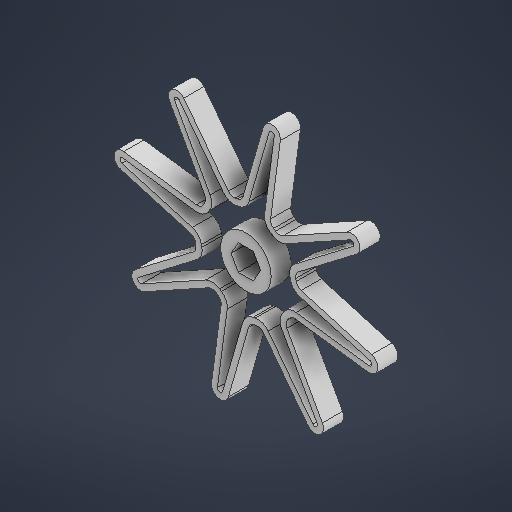
# Autodesk Inventor part: molde star
Saved by Autodesk Inventor 2025 (Build 290162010, 162A)
## iProperties
Created: 2025-01-06
Part Number: molde star
Material: Genérico
Document SubType Name: Modeling
Designer: Win-10
Density: 1 g/cm^3
Appearance: Padrão
Author: Win-10
Autodesk Inventor part; units mm, degrees
ref_plane "YZ Plane" through (0, 0, 0) normal (1, 0, 0) x (0, 1, 0)
ref_plane "XZ Plane" through (0, 0, 0) normal (0, 1, 0) x (-1, 0, 0)
ref_plane "XY Plane" through (0, 0, 0) normal (0, 0, 1) x (1, 0, 0)
sketch "Esboço1" plane through (0, 0, 0) normal (0, 0, 1) x (1, 0, 0)
  line L0 (51.4739, 35.1611) -> (19.7673, 17.6332) projected
  arc A0 (12.9851, 18.0371) -> (19.7673, 17.6332) centre (16.6951, 23.1906) ccw projected
  line L1 (12.9851, 18.0371) -> (12.0737, 18.6595) projected
  arc A1 (9.229, 24.8295) -> (12.0737, 18.6595) centre (15.5233, 23.9908) ccw projected
  line L2 (9.229, 24.8295) -> (14.0142, 60.741) projected
  arc A2 (14.0142, 60.741) -> (11.5349, 61.2602) centre (12.7553, 60.9087) ccw projected
  line L3 (11.5349, 61.2602) -> (1.509, 26.4462) projected
  arc A3 (-3.5723, 21.936) -> (1.509, 26.4462) centre (-4.593, 28.2035) ccw projected
  line L4 (-3.5723, 21.936) -> (-4.6569, 21.7316) projected
  arc A4 (-11.0312, 24.083) -> (-4.6569, 21.7316) centre (-5.9874, 27.9407) ccw projected
  line L5 (-11.0312, 24.083) -> (-33.0408, 52.8599) projected
  arc A5 (-33.0408, 52.8599) -> (-35.1611, 51.4739) centre (-34.0496, 52.0884) ccw projected
  line L6 (-35.1611, 51.4739) -> (-17.6332, 19.7673) projected
  arc A6 (-18.0371, 12.9851) -> (-17.6332, 19.7673) centre (-23.1906, 16.6951) ccw projected
  line L7 (-18.0371, 12.9851) -> (-18.6595, 12.0737) projected
  arc A7 (-24.8295, 9.229) -> (-18.6595, 12.0737) centre (-23.9908, 15.5233) ccw projected
  line L8 (-24.8295, 9.229) -> (-60.741, 14.0142) projected
  arc A8 (-60.741, 14.0142) -> (-61.2602, 11.5349) centre (-60.9087, 12.7553) ccw projected
  line L9 (-61.2602, 11.5349) -> (-26.4462, 1.509) projected
  arc A9 (-21.936, -3.5723) -> (-26.4462, 1.509) centre (-28.2035, -4.593) ccw projected
  line L10 (-21.936, -3.5723) -> (-21.7316, -4.6569) projected
  arc A10 (-24.083, -11.0312) -> (-21.7316, -4.6569) centre (-27.9407, -5.9874) ccw projected
  line L11 (-24.083, -11.0312) -> (-52.8599, -33.0408) projected
  arc A11 (-52.8599, -33.0408) -> (-51.4739, -35.1611) centre (-52.0884, -34.0496) ccw projected
  line L12 (-51.4739, -35.1611) -> (-19.7673, -17.6332) projected
  arc A12 (-12.9851, -18.0371) -> (-19.7673, -17.6332) centre (-16.6951, -23.1906) ccw projected
  line L13 (-12.9851, -18.0371) -> (-12.0737, -18.6595) projected
  arc A13 (-9.229, -24.8295) -> (-12.0737, -18.6595) centre (-15.5233, -23.9908) ccw projected
  line L14 (-9.229, -24.8295) -> (-14.0142, -60.741) projected
  arc A14 (-14.0142, -60.741) -> (-11.5349, -61.2602) centre (-12.7553, -60.9087) ccw projected
  line L15 (-11.5349, -61.2602) -> (-1.509, -26.4462) projected
  arc A15 (3.5723, -21.936) -> (-1.509, -26.4462) centre (4.593, -28.2035) ccw projected
  line L16 (3.5723, -21.936) -> (4.6569, -21.7316) projected
  arc A16 (11.0312, -24.083) -> (4.6569, -21.7316) centre (5.9874, -27.9407) ccw projected
  line L17 (11.0312, -24.083) -> (33.0408, -52.8599) projected
  arc A17 (33.0408, -52.8599) -> (35.1611, -51.4739) centre (34.0496, -52.0884) ccw projected
  line L18 (35.1611, -51.4739) -> (17.6332, -19.7673) projected
  arc A18 (18.0371, -12.9851) -> (17.6332, -19.7673) centre (23.1906, -16.6951) ccw projected
  line L19 (18.0371, -12.9851) -> (18.6595, -12.0737) projected
  arc A19 (24.8295, -9.229) -> (18.6595, -12.0737) centre (23.9908, -15.5233) ccw projected
  line L20 (24.8295, -9.229) -> (60.741, -14.0142) projected
  arc A20 (60.741, -14.0142) -> (61.2602, -11.5349) centre (60.9087, -12.7553) ccw projected
  line L21 (61.2602, -11.5349) -> (26.4462, -1.509) projected
  arc A21 (21.936, 3.5723) -> (26.4462, -1.509) centre (28.2035, 4.593) ccw projected
  line L22 (21.936, 3.5723) -> (21.7316, 4.6569) projected
  arc A22 (24.083, 11.0312) -> (21.7316, 4.6569) centre (27.9407, 5.9874) ccw projected
  line L23 (24.083, 11.0312) -> (52.8599, 33.0408) projected
  arc A23 (52.8599, 33.0408) -> (51.4739, 35.1611) centre (52.0884, 34.0496) ccw projected
  line L24 (54.6824, 30.6579) -> (25.9055, 8.6483)
  arc A24 (25.9055, 8.6483) -> (24.6718, 5.2548) centre (27.9407, 5.9874) ccw
  line L25 (24.6718, 5.2548) -> (24.8921, 4.0855)
  arc A25 (24.8921, 4.0855) -> (27.2764, 1.3738) centre (28.2035, 4.593) ccw
  line L26 (27.2764, 1.3738) -> (62.0904, -8.6521)
  arc A26 (60.3447, -16.9879) -> (62.0904, -8.6521) centre (60.9087, -12.7553) ccw
  line L27 (60.3447, -16.9879) -> (24.4332, -12.2027)
  arc A27 (24.4332, -12.2027) -> (21.1613, -13.7298) centre (23.9908, -15.5233) ccw
  line L28 (21.1613, -13.7298) -> (20.4903, -14.7125)
  arc A28 (20.4903, -14.7125) -> (20.2587, -18.3159) centre (23.1906, -16.6951) ccw
  line L29 (20.2587, -18.3159) -> (37.7866, -50.0225)
  arc A29 (30.6579, -54.6824) -> (37.7866, -50.0225) centre (34.0496, -52.0884) ccw
  line L30 (30.6579, -54.6824) -> (8.6483, -25.9055)
  arc A30 (8.6483, -25.9055) -> (5.2548, -24.6718) centre (5.9874, -27.9407) ccw
  line L31 (5.2548, -24.6718) -> (4.0855, -24.8921)
  arc A31 (4.0855, -24.8921) -> (1.3738, -27.2764) centre (4.593, -28.2035) ccw
  line L32 (1.3738, -27.2764) -> (-8.6521, -62.0904)
  arc A32 (-16.9879, -60.3447) -> (-8.6521, -62.0904) centre (-12.7553, -60.9087) ccw
  line L33 (-16.9879, -60.3447) -> (-12.2027, -24.4332)
  arc A33 (-12.2027, -24.4332) -> (-13.7298, -21.1613) centre (-15.5233, -23.9908) ccw
  line L34 (-13.7298, -21.1613) -> (-14.7125, -20.4903)
  arc A34 (-14.7125, -20.4903) -> (-18.3159, -20.2587) centre (-16.6951, -23.1906) ccw
  line L35 (-18.3159, -20.2587) -> (-50.0225, -37.7866)
  arc A35 (-54.6824, -30.6579) -> (-50.0225, -37.7866) centre (-52.0884, -34.0496) ccw
  line L36 (-54.6824, -30.6579) -> (-25.9055, -8.6483)
  arc A36 (-25.9055, -8.6483) -> (-24.6718, -5.2548) centre (-27.9407, -5.9874) ccw
  line L37 (-24.6718, -5.2548) -> (-24.8921, -4.0855)
  arc A37 (-24.8921, -4.0855) -> (-27.2764, -1.3738) centre (-28.2035, -4.593) ccw
  line L38 (-27.2764, -1.3738) -> (-62.0904, 8.6521)
  arc A38 (-60.3447, 16.9879) -> (-62.0904, 8.6521) centre (-60.9087, 12.7553) ccw
  line L39 (-60.3447, 16.9879) -> (-24.4332, 12.2027)
  arc A39 (-24.4332, 12.2027) -> (-21.1613, 13.7298) centre (-23.9908, 15.5233) ccw
  line L40 (-21.1613, 13.7298) -> (-20.4903, 14.7125)
  arc A40 (-20.4903, 14.7125) -> (-20.2587, 18.3159) centre (-23.1906, 16.6951) ccw
  line L41 (-20.2587, 18.3159) -> (-37.7866, 50.0225)
  arc A41 (-30.6579, 54.6824) -> (-37.7866, 50.0225) centre (-34.0496, 52.0884) ccw
  line L42 (-30.6579, 54.6824) -> (-8.6483, 25.9055)
  arc A42 (-8.6483, 25.9055) -> (-5.2548, 24.6718) centre (-5.9874, 27.9407) ccw
  line L43 (-5.2548, 24.6718) -> (-4.0855, 24.8921)
  arc A43 (-4.0855, 24.8921) -> (-1.3738, 27.2764) centre (-4.593, 28.2035) ccw
  line L44 (-1.3738, 27.2764) -> (8.6521, 62.0904)
  arc A44 (16.9879, 60.3447) -> (8.6521, 62.0904) centre (12.7553, 60.9087) ccw
  line L45 (16.9879, 60.3447) -> (12.2027, 24.4332)
  arc A45 (12.2027, 24.4332) -> (13.7298, 21.1613) centre (15.5233, 23.9908) ccw
  line L46 (13.7298, 21.1613) -> (14.7125, 20.4903)
  arc A46 (14.7125, 20.4903) -> (18.3159, 20.2587) centre (16.6951, 23.1906) ccw
  line L47 (18.3159, 20.2587) -> (50.0225, 37.7866)
  arc A47 (54.6824, 30.6579) -> (50.0225, 37.7866) centre (52.0884, 34.0496) ccw
  circle A48 centre (0, 0) radius 12.5
  line L48 (7.3323, 0) -> (3.6662, -6.35)
  line L49 (3.6662, -6.35) -> (-3.6662, -6.35)
  line L50 (-3.6662, -6.35) -> (-7.3323, 0)
  line L51 (-7.3323, 0) -> (-3.6662, 6.35)
  line L52 (-3.6662, 6.35) -> (3.6662, 6.35)
  line L53 (3.6662, 6.35) -> (7.3323, 0)
  dimension "d0" = 25
  dimension "d1" = 12.7
  dimension "d2" = 36.2289
  dimension "d3" = 4.27
  dimension "d4" = 3.35
  dimension "d6" = 3.6108
  dimension "d7" = 3.6108
  dimension "d8" = 3.6108
  dimension "d9" = 3.6108
  dimension "d10" = 3.6034
  dimension "d11" = 3.6108
  dimension "d12" = 3.6034
  constraints: 60 end point, 48 point on circle, 25 centre point, 23 equal length, 22 equal radius, 16 tangent, 2 coincident, 1 horizontal, 14 other
  measures "d0" diameter of A48
  measures "d1" distance between parallel lines of L49 L52
  measures "d2" distance of L42.start L42.end
  measures "d3" radius of A41
  measures "d4" radius of A42
  measures "d6" distance of L45.end L46.start
  measures "d7" distance of L24.end L25.start
  measures "d8" distance of L27.end L28.start
  measures "d9" distance of L30.end L31.start
  measures "d10" horizontal distance of L35.start L34.end
  measures "d11" distance of L38.start L37.end
  measures "d12" vertical distance of L41.start L40.end
extrude "Extrusão1" add sketch "Esboço1" along normal blind 10
